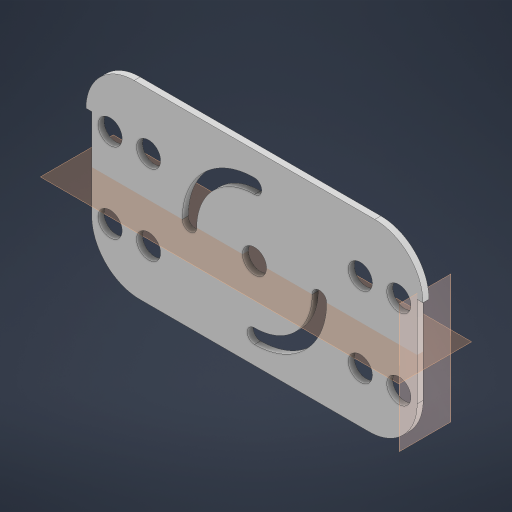
# Autodesk Inventor part: Plate
Saved by Autodesk Inventor 2024 (Build 280153000, 153)
## iProperties
Created: 2024-02-01
Part Number: Plate
Material: Generic
Document SubType Name: Modeling
Designer: calvi
Density: 1 g/cm^3
Appearance: Default
Author: calvi
Autodesk Inventor part; units mm, degrees
ref_plane "YZ Plane" through (0, 0, 0) normal (1, 0, 0) x (0, 1, 0)
ref_plane "XZ Plane" through (0, 0, 0) normal (0, 1, 0) x (-1, 0, 0)
ref_plane "XY Plane" through (0, 0, 0) normal (0, 0, 1) x (1, 0, 0)
sketch "Sketch3" plane through (0, 0, 0) normal (0, 0, 1) x (1, 0, 0)
  line L0 (0, 0) -> (177.8, 0)
  line L1 (177.8, 0) -> (177.8, 101.6)
  line L2 (177.8, 101.6) -> (0, 101.6)
  line L3 (0, 101.6) -> (0, 0)
  arc A0 (25.4, 101.6) -> (0, 76.2) centre (25.4, 76.2) ccw
  arc A1 (177.8, 76.2) -> (152.4, 101.6) centre (152.4, 76.2) ccw
  arc A2 (152.4, 0) -> (177.8, 25.4) centre (152.4, 25.4) ccw
  arc A3 (0, 25.4) -> (25.4, 0) centre (25.4, 25.4) ccw
  circle A4 centre (88.9, 50.8) radius 6.35
  arc A5 (88.9, 85.09) -> (54.61, 50.8) centre (88.9, 50.8) ccw construction
  arc A6 (88.9, 88.9) -> (50.8, 50.8) centre (88.9, 50.8) ccw
  arc A7 (88.9, 81.28) -> (58.42, 50.8) centre (88.9, 50.8) ccw
  arc A8 (88.9, 81.28) -> (88.9, 88.9) centre (88.9, 85.09) ccw
  arc A9 (50.8, 50.8) -> (58.42, 50.8) centre (54.61, 50.8) ccw
  line L4 (88.9, 50.8) -> (54.61, 50.8) construction
  line L5 (88.9, 50.8) -> (88.9, 85.09) construction
  arc A10 (88.9, 20.32) -> (119.38, 50.8) centre (88.9, 50.8) ccw
  line L6 (88.9, 50.8) -> (123.19, 50.8) construction
  arc A11 (88.9, 16.51) -> (123.19, 50.8) centre (88.9, 50.8) ccw construction
  arc A12 (127, 50.8) -> (119.38, 50.8) centre (123.19, 50.8) ccw
  arc A13 (88.9, 12.7) -> (127, 50.8) centre (88.9, 50.8) ccw
  arc A14 (88.9, 20.32) -> (88.9, 12.7) centre (88.9, 16.51) ccw
  dimension "d20" = 177.8
  dimension "d21" = 101.6
  dimension "d22" = 50.8
  dimension "d23" = 50.8
  dimension "d24" = 50.8
  dimension "d25" = 50.8
  dimension "d26" = 12.7
  dimension "d27" = 50.8
  dimension "d28" = 88.9
  dimension "d29" = 34.29
  dimension "d30" = 90
  dimension "d31" = 7.62
  dimension "d34" = 360
  constraints: 28 point on circle, 15 centre point, 14 end point, 12 tangent, 8 point on line, 2 parallel, 1 coincident, 1 horizontal, 1 perpendicular, 1 vertical, 27 other
  measures "d20" distance of L2.end L1.end
  measures "d21" distance of L1.end L0.end
  measures "d22" diameter of A0
  measures "d23" diameter of A1
  measures "d24" diameter of A2
  measures "d25" diameter of A3
  measures "d26" diameter of A4
  measures "d27" distance from line of L0 A4.centre
  measures "d28" distance from line of L1 A4.centre
  measures "d29" radius of A5
  measures "d30" angle of L5 L4
  measures "d31" diameter of A9
extrude "Extrusion3" add sketch "Sketch3" against normal blind 3.175 contours A3 L3 A0 L2 A1 L1 A2 L0
ref_plane "Work Plane1" through (25.4, 50.8, 0) normal (0, 1, 0) x (1, 0, 0)
sketch "Sketch4" plane through (0, 0, 0) normal (0, 0, 1) x (1, 0, 0)
  line L0 (0, 76.2) -> (0, 25.4) projected
  line L1 (0, 50.8) -> (177.8, 50.8)
  line L2 (177.8, 76.2) -> (177.8, 25.4) projected
  line L3 (152.4, 101.6) -> (25.4, 101.6) projected
  line L4 (88.9, 101.6) -> (88.9, 0)
  circle A0 centre (12.7, 71.882) radius 6.35
  circle A1 centre (33.02, 71.882) radius 6.35
  line L5 (0, 25.4) -> (0, 76.2)
  circle A2 centre (12.7, 29.718) radius 6.35
  circle A3 centre (33.02, 29.718) radius 6.35
  circle A4 centre (165.1, 71.882) radius 6.35
  circle A5 centre (144.78, 71.882) radius 6.35
  circle A6 centre (165.1, 29.718) radius 6.35
  circle A7 centre (144.78, 29.718) radius 6.35
  point P0 (0, 0)
  dimension "d39" = 12.7
  dimension "d40" = 12.7
  dimension "d41" = 20.32
  dimension "d42" = 12.7
  dimension "d43" = 21.082
  constraints: 8 centre point, 8 symmetric about line, 6 end point, 3 midpoint, 1 horizontal alignment, 1 vertical, 6 other
  measures "d39" diameter of A0
  measures "d40" diameter of A1
  measures "d41" distance of A1.centre A0.centre
  measures "d42" distance from line of L0 A0.centre
  measures "d43" distance from line of L1 A0.centre
extrude "Extrusion4" cut sketch "Sketch4" against normal blind 25.4
sketch "Sketch5" plane through (177.8, 25.4, 0) normal (1, 0, 0) x (0, 0, -1)
  line L0 (3.175, 50.8) -> (3.175, 76.2) projected
  line L1 (0, -25.4) -> (3.175, -25.4)
  line L2 (3.175, -25.4) -> (3.175, 50.8)
  line L3 (3.175, 50.8) -> (0, 50.8)
  line L4 (0, 50.8) -> (0, -25.4)
  constraints: 8 end point, 2 parallel, 1 horizontal, 1 perpendicular
extrude "Extrusion5" cut sketch "Sketch5" against normal blind 3.048
sketch "Sketch6" plane through (0, 25.4, 0) normal (-1, 0, 0) x (0, 0, 1)
  line L0 (0, 50.8) -> (-3.175, 50.8) projected
  line L1 (-3.175, 50.8) -> (0, 50.8)
  line L2 (0, 50.8) -> (0, -25.4)
  line L3 (0, -25.4) -> (-3.175, -25.4)
  line L4 (-3.175, -25.4) -> (-3.175, 50.8)
  constraints: 8 end point, 2 parallel, 1 horizontal, 1 perpendicular
extrude "Extrusion6" cut sketch "Sketch6" against normal blind 3.048
sketch "Sketch7" plane through (25.4, 0, 0) normal (0, -1, 0) x (1, 0, 0)
  line L0 (-22.352, -3.175) -> (-22.352, 0) projected
  line L1 (127, -3.175) -> (152.4, -3.175) projected
  line L2 (-22.352, 0) -> (149.352, 0)
  line L3 (149.352, 0) -> (149.352, -3.175)
  line L4 (149.352, -3.175) -> (-22.352, -3.175)
  line L5 (-22.352, -3.175) -> (-22.352, 0)
  point P0 (-25.4, 0)
  point P1 (149.352, -1.5875)
  dimension "d50" = 171.704
  constraints: 8 end point, 2 parallel, 1 horizontal, 1 midpoint, 1 perpendicular, 1 point on line
  measures "d50" distance from line of point (149.352, -1.587) L0
extrude "Extrusion7" cut sketch "Sketch7" against normal blind 3.048
sketch "Sketch8" plane through (0, 0, 0) normal (0, 0, 1) x (1, 0, 0)
  arc A0 (3.048, 28.448) -> (28.448, 3.048) centre (28.448, 28.448) ccw
  arc A1 (149.352, 3.048) -> (174.752, 28.448) centre (149.352, 28.448) ccw
  line L0 (174.752, 13.3357) -> (174.752, 76.2) projected
  line L1 (13.3357, 3.048) -> (164.4643, 3.048) projected
  line L2 (3.048, 76.2) -> (3.048, 13.3357) projected
  line L3 (3.048, 28.448) -> (3.048, 3.048)
  line L4 (3.048, 3.048) -> (28.448, 3.048)
  line L5 (174.752, 28.448) -> (174.752, 3.048)
  line L6 (174.752, 3.048) -> (149.352, 3.048)
  point P0 (0, 0)
  point P1 (3.048, 13.3357)
  dimension "d53" = 50.8
  dimension "d54" = 50.8
  constraints: 8 end point, 7 tangent, 6 point on line, 4 point on circle, 2 centre point, 1 collinear, 1 perpendicular
  measures "d53" diameter of A0
  measures "d54" diameter of A1
extrude "Extrusion8" cut sketch "Sketch8" against normal through all
ref_plane "Work Plane2" through (174.752, 25.4, 0) normal (1, 0, 0) x (0, 0, -1)
body "Solid2"
